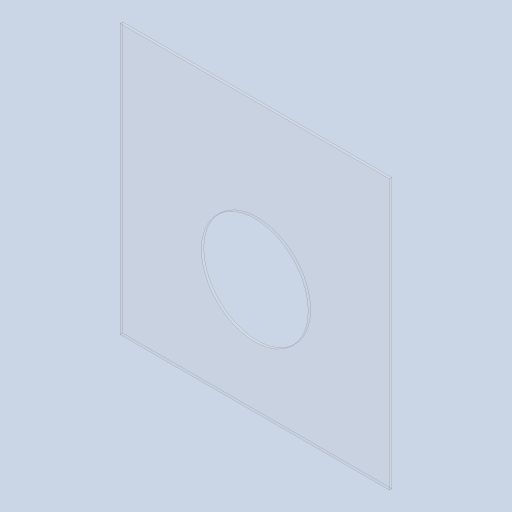
# Autodesk Inventor part: cage_wall
Saved by Autodesk Inventor 2024.4 (Build 284460000, 460)
## iProperties
Created: 2026-03-25
Part Number: cage_wall
Material: Generic
Document SubType Name: Modeling
Designer: tooles01
Density: 1 g/cm^3
Appearance: Clear - Light
Author: tooles01
Autodesk Inventor part; units mm, degrees
ref_plane "YZ Plane" through (0, 0, 0) normal (1, 0, 0) x (0, 1, 0)
ref_plane "XZ Plane" through (0, 0, 0) normal (0, 1, 0) x (-1, 0, 0)
ref_plane "XY Plane" through (0, 0, 0) normal (0, 0, 1) x (1, 0, 0)
sketch "Sketch1" plane through (0, 0, 0) normal (0, 0, 1) x (1, 0, 0)
  line L0 (-3.4369, 182.883) -> (106.5631, 182.883)
  line L1 (106.5631, 182.883) -> (106.5631, 42.883)
  line L2 (106.5631, 42.883) -> (-3.4369, 42.883)
  line L3 (-3.4369, 42.883) -> (-3.4369, 182.883)
  circle A0 centre (51.5631, 76.8468) radius 15.875
  line L4 (-3.4369, 122.883) -> (106.5631, 122.883)
  line L5 (91.5631, 122.883) -> (91.5631, 42.883)
  line L6 (11.5631, 122.883) -> (11.5631, 42.883)
  point P0 (0, 0)
  point P1 (51.5631, 42.883)
  dimension "d0" = 140
  dimension "d1" = 110
  dimension "d2" = 31.75
  dimension "d5" = 80
  dimension "d6" = 15
  dimension "d7" = 15
  constraints: 14 end point, 6 point on line, 3 perpendicular, 1 centre point, 1 horizontal, 1 midpoint, 1 vertical alignment, 1 other
  measures "d0" distance of L2.end L0.start
  measures "d1" distance of L0.start L0.end
  measures "d2" diameter of A0
  measures "d5" distance between parallel lines of L2 L4
  measures "d6" distance between parallel lines of L3 L6
  measures "d7" distance between parallel lines of L1 L5
extrude "Extrusion1" add sketch "Sketch1" against normal blind 0.7 contours L4 L5 L2 L6
equation "\"d7\" = d6"
body "Solid1"
